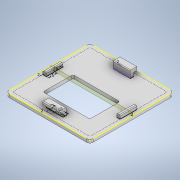
# Autodesk Inventor part: 180caseTop
Saved by Autodesk Inventor 2022 (Build 260153000, 153)
## iProperties
Created: 2022-03-13
Part Number: 180caseTop
Material: Generic
Document SubType Name: Modeling
Designer: maksym
Density: 1 g/cm^3
Appearance: Default
Author: maksym
Autodesk Inventor part; units mm, degrees
ref_plane "YZ Plane" through (0, 0, 0) normal (1, 0, 0) x (0, 1, 0)
ref_plane "XZ Plane" through (0, 0, 0) normal (0, 1, 0) x (-1, 0, 0)
ref_plane "XY Plane" through (0, 0, 0) normal (0, 0, 1) x (1, 0, 0)
sketch "Sketch1" plane through (0, 0, 0) normal (0, 1, 0) x (-1, 0, 0)
  line L0 (0, 0) -> (50, 0)
  line L1 (50, 0) -> (50, -50)
  line L2 (50, -50) -> (0, -50)
  line L3 (0, -50) -> (0, 0)
  dimension "d0" = 50
  dimension "d1" = 50
  constraints: 8 end point, 2 parallel, 1 horizontal, 1 perpendicular
  measures "d0" distance of L1.end L2.end
  measures "d1" distance of L0.end L1.end
extrude "Extrusion1" add sketch "Sketch1" along normal blind 2
fillet "Fillet1" radius 2 4 edges at (0, 1, 0) (0, 1, -50) (-50, 1, 0) (-50, 1, -50)
sketch "Sketch2" plane through (0, 2, 0) normal (0, 1, 0) x (1, 0, 0)
  line L0 (-48, 2) -> (-2, 2) construction
  line L1 (-2, 2) -> (-2, 48) construction
  line L2 (-2, 48) -> (-48, 48) construction
  line L3 (-48, 48) -> (-48, 2) construction
  line L4 (-48, 0) -> (-2, 0) projected
  line L5 (-50, 48) -> (-50, 2) projected
  line L6 (-2, 50) -> (-48, 50) projected
  line L7 (0, 2) -> (0, 48) projected
  line L8 (-25, 2) -> (-25, 6) construction
  line L9 (-25, 4) -> (-20, 4)
  line L10 (-20, 4) -> (-20, 6)
  line L11 (-20, 6) -> (-30, 6)
  line L12 (-30, 6) -> (-30, 4)
  line L13 (-30, 4) -> (-25, 4)
  line L14 (-48, 25) -> (-46, 25) construction
  line L15 (-46, 25) -> (-46, 20)
  line L16 (-46, 20) -> (-48, 20)
  line L17 (-46, 25) -> (-46, 30)
  line L18 (-46, 30) -> (-48, 30)
  line L19 (-48, 20) -> (-48, 30)
  line L20 (-4, 25) -> (-4, 20)
  line L21 (-4, 20) -> (-2, 20)
  line L22 (-4, 25) -> (-4, 30)
  line L23 (-4, 30) -> (-2, 30)
  line L24 (-2, 20) -> (-2, 30)
  line L25 (-25, 48) -> (-25, 44) construction
  line L26 (-25, 46) -> (-20, 46)
  line L27 (-20, 46) -> (-20, 44)
  line L28 (-20, 44) -> (-30, 44)
  line L29 (-30, 44) -> (-30, 46)
  line L30 (-30, 46) -> (-25, 46)
  point P0 (0, 0)
  dimension "d5" = 2
  dimension "d6" = 2
  dimension "d7" = 2
  dimension "d8" = 2
  dimension "d9" = 4
  dimension "d10" = 5
  dimension "d11" = 10
  dimension "d12" = 2
  dimension "d13" = 5
  dimension "d14" = 5
  constraints: 54 end point, 12 symmetric about line, 7 perpendicular, 4 point on line, 3 equal length, 3 horizontal, 3 midpoint, 3 vertical
  measures "d5" distance between parallel lines of L4 L0
  measures "d6" distance between parallel lines of L5 L3
  measures "d7" distance between parallel lines of L6 L2
  measures "d8" distance between parallel lines of L7 L1
  measures "d9" distance of L8.start L8.end
  measures "d10" distance of L9.start L9.end
  measures "d11" distance of L10.end L11.end
  measures "d12" distance of L14.start L14.end
  measures "d13" distance of L14.end L15.end
  measures "d14" distance of L14.end L17.end
extrude "Extrusion2" add sketch "Sketch2" along normal blind 2 contours L15 L16 L19 L18 L17 | L22 L23 L24 L21 L20
extrude "Extrusion3" add sketch "Sketch2" along normal blind 4.1 contours L13 L12 L11 L10 L9 | L26 L27 L28 L29 L30
sketch "Sketch3" plane through (-20, 2, -46) normal (0, 0, -1) x (-1, 0, 0)
  line L0 (10, 4.1) -> (0, 4.1) projected
  line L1 (0, 4.1) -> (10, 4.1)
  line L2 (10, 4.1) -> (10, 2.1)
  line L3 (10, 2.1) -> (0, 2.1)
  line L4 (0, 2.1) -> (0, 4.1)
  point P0 (-20, -2)
  dimension "d19" = 10
  dimension "d20" = 2
  constraints: 8 end point, 2 parallel, 1 horizontal, 1 perpendicular
  measures "d19" distance of L2.end L3.end
  measures "d20" distance of L1.end L2.end
extrude "Extrusion4" add sketch "Sketch3" along normal blind 2
fillet "Fillet2" radius 0.5 1 edges at (-25, 4.1, -48)
ref_plane "Work Plane1" through (-46, 4, -25) normal (0, 0, -1) x (1, 0, 0)
mirror "Mirror1" about plane through (-46, 4, -25) normal (0, 0, -1) of "Extrusion4"
fillet "Fillet3" radius 0.5 1 edges at (-25, 4.1, -2)
fillet "Fillet4" radius 0.5 7 edges at (-2, 4, -25) (-4, 4, -25) (-46, 4, -25) (-48, 4, -25) (-25, 6.1, -2) (-25, 6.1, -6) (-25, 6.1, -44)
sketch "Sketch4" plane through (0, 2, 0) normal (0, 1, 0) x (1, 0, 0)
  line L0 (-30, 2.5) -> (-20, 2.5) projected
  line L1 (-25, 2.5) -> (-25, 49.5156) construction
  line L2 (-30, 46) -> (-20, 46) projected
  line L3 (-11, 11) -> (-39, 11)
  line L4 (-39, 11) -> (-39, 29)
  line L5 (-39, 29) -> (-11, 29)
  line L6 (-11, 29) -> (-11, 11)
  line L7 (-11, 11) -> (-39, 29) construction
  line L8 (-39, 11) -> (-11, 29) construction
  line L9 (-48, 0) -> (-2, 0) projected
  point P0 (0, 0)
  point P1 (-25, 20)
  dimension "d26" = 28
  dimension "d27" = 18
  dimension "d28" = 20
  constraints: 14 end point, 3 midpoint, 2 parallel, 2 perpendicular, 1 horizontal, 1 point on line
  measures "d26" distance of L4.end L5.end
  measures "d27" distance of L3.end L4.end
  measures "d28" distance from line of L9 point (-25, 20)
extrude "Extrusion5" cut sketch "Sketch4" against normal blind 2
fillet "Fillet5" radius 1 4 edges at (-39, 1, -11) (-11, 1, -11) (-11, 1, -29) (-39, 1, -29)
body "Solid1"
